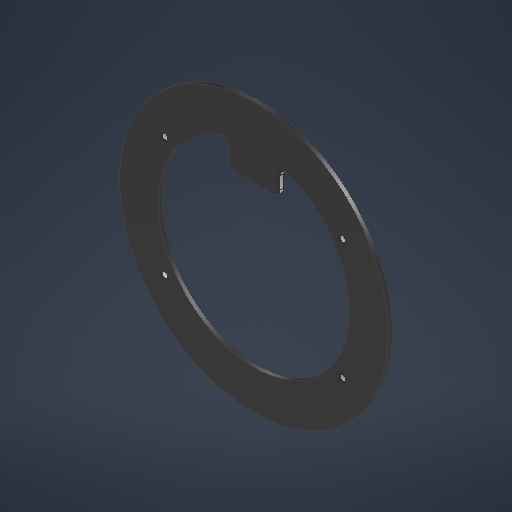
# Autodesk Inventor part: IR Board
Saved by Autodesk Inventor 2026.1 (Build 301233020, 233B)
## iProperties
Created: 2025-11-27
Part Number: IR Board
Material: Generic
Document SubType Name: Modeling
Designer: Bahaa
Density: 1 g/cm^3
Appearance: Default
Mass: 13.7907 g
Surface Area: 152.933 cm^2
Volume: 13.7907 cm^3
Author: Bahaa
Autodesk Inventor part; units mm, degrees
ref_plane "YZ Plane" through (0, 0, 0) normal (1, 0, 0) x (0, 1, 0)
ref_plane "XZ Plane" through (0, 0, 0) normal (0, 1, 0) x (-1, 0, 0)
ref_plane "XY Plane" through (0, 0, 0) normal (0, 0, 1) x (1, 0, 0)
sketch "Sketch1" plane through (0, 0, 0) normal (0, 1, 0) x (-1, 0, 0)
  circle A0 centre (0, 0) radius 65
  line L0 (0, 0) -> (65, 0) construction
  line L1 (0, 0) -> (0, -65) construction
  circle A1 centre (0, 0) radius 46.25
  line L2 (0, 46.25) -> (0, 31.25)
  line L3 (0, 31.25) -> (-34.0955, 31.25)
  line L4 (0, 31.25) -> (34.0955, 31.25)
  line L5 (0, 0) -> (65, 0) construction
  line L6 (0, 0) -> (-46.25, 0) construction
  circle A2 centre (29, 43) radius 1.35
  circle A3 centre (-29, 43) radius 1.35
  circle A4 centre (29, -43) radius 1.35
  circle A5 centre (-29, -43) radius 1.35
  circle A6 centre (-43, 29) radius 1.35
  circle A7 centre (-43, -29) radius 1.35
  circle A8 centre (43, 29) radius 1.35
  circle A9 centre (43, -29) radius 1.35
  circle A10 centre (-29, -43) radius 1.35
  circle A11 centre (29, -43) radius 1.35
  circle A12 centre (-29, 43) radius 1.35
  circle A13 centre (29, 43) radius 1.35
  circle A14 centre (43, -29) radius 1.35
  circle A15 centre (43, 29) radius 1.35
  circle A16 centre (-43, -29) radius 1.35
  circle A17 centre (-43, 29) radius 1.35
  line L7 (12.5, 46.25) -> (-12.5, 46.25)
  line L8 (-12.5, 46.25) -> (-12.5, 31.25)
  line L9 (-12.5, 31.25) -> (12.5, 31.25)
  line L10 (12.5, 31.25) -> (12.5, 46.25)
  line L11 (12.5, 46.25) -> (-12.5, 31.25) construction
  line L12 (-12.5, 46.25) -> (12.5, 31.25) construction
  point P0 (0, -46.25)
  point P1 (0, 38.75)
  point P2 (-12.5, 44.5288)
  point P3 (12.5, 44.5288)
  dimension "d0" = 130
  dimension "d18" = 92.5
  dimension "d21" = 62.5
  dimension "d29" = 86
  dimension "d30" = 29
  dimension "d31" = 2.7
  dimension "d47" = 360
  dimension "d49" = 25
  constraints: 26 end point, 18 centre point, 6 coincident, 6 point on circle, 5 symmetric about line, 4 horizontal, 3 midpoint, 2 parallel, 2 perpendicular, 2 point on line, 2 vertical, 1 vertical alignment, 38 other
  measures "d0" diameter of A0
  measures "d18" diameter of A1
  measures "d21" diameter of L3 L0
  measures "d29" diameter of point (29, 43) L0
  measures "d30" horizontal distance of point (0, 0) point (29, 43)
  measures "d31" diameter of A2
  measures "d49" distance of L9.end L8.end
extrude "Extrusion1" add sketch "Sketch1" along normal blind 2 contours A0 | L10 L4 L2 A1 | A1 L7 L10 | L8 L7 A1 | A1 L2 L3 L8 | A2 | A3 | A4 | A5
sketch "Sketch2" plane through (0, 0, 0) normal (0, -1, 0) x (1, 0, 0)
  circle A0 centre (0, 0) radius 65 construction
  line L0 (-4, 55) -> (4, 55)
  line L1 (4, 55) -> (4, 61)
  line L2 (-4, 61) -> (-4, 55)
  line L3 (-4, 55) -> (4, 61) construction
  line L4 (4, 55) -> (-4, 61) construction
  line L5 (0, 0) -> (0, 71.2779) construction
  arc A1 (4, 61) -> (-4, 61) centre (0, 61) ccw
  line L6 (-24.7431, 49.2826) -> (-17.3521, 52.3441)
  line L7 (-17.3521, 52.3441) -> (-19.6482, 57.8874)
  line L8 (-27.0392, 54.8259) -> (-24.7431, 49.2826)
  line L9 (-24.7431, 49.2826) -> (-19.6482, 57.8874) construction
  line L10 (-17.3521, 52.3441) -> (-27.0392, 54.8259) construction
  arc A2 (-19.6482, 57.8874) -> (-27.0392, 54.8259) centre (-23.3437, 56.3567) ccw
  line L11 (-41.7193, 36.0624) -> (-36.0624, 41.7193)
  line L12 (-36.0624, 41.7193) -> (-40.3051, 45.9619)
  line L13 (-45.9619, 40.3051) -> (-41.7193, 36.0624)
  line L14 (-41.7193, 36.0624) -> (-40.3051, 45.9619) construction
  line L15 (-36.0624, 41.7193) -> (-45.9619, 40.3051) construction
  arc A3 (-40.3051, 45.9619) -> (-45.9619, 40.3051) centre (-43.1335, 43.1335) ccw
  line L16 (-52.3441, 17.3521) -> (-49.2826, 24.7431)
  line L17 (-49.2826, 24.7431) -> (-54.8259, 27.0392)
  line L18 (-57.8874, 19.6482) -> (-52.3441, 17.3521)
  line L19 (-52.3441, 17.3521) -> (-54.8259, 27.0392) construction
  line L20 (-49.2826, 24.7431) -> (-57.8874, 19.6482) construction
  arc A4 (-54.8259, 27.0392) -> (-57.8874, 19.6482) centre (-56.3567, 23.3437) ccw
  line L21 (-55, -4) -> (-55, 4)
  line L22 (-55, 4) -> (-61, 4)
  line L23 (-61, -4) -> (-55, -4)
  line L24 (-55, -4) -> (-61, 4) construction
  line L25 (-55, 4) -> (-61, -4) construction
  arc A5 (-61, 4) -> (-61, -4) centre (-61, 0) ccw
  line L26 (-49.2826, -24.7431) -> (-52.3441, -17.3521)
  line L27 (-52.3441, -17.3521) -> (-57.8874, -19.6482)
  line L28 (-54.8259, -27.0392) -> (-49.2826, -24.7431)
  line L29 (-49.2826, -24.7431) -> (-57.8874, -19.6482) construction
  line L30 (-52.3441, -17.3521) -> (-54.8259, -27.0392) construction
  arc A6 (-57.8874, -19.6482) -> (-54.8259, -27.0392) centre (-56.3567, -23.3437) ccw
  line L31 (-36.0624, -41.7193) -> (-41.7193, -36.0624)
  line L32 (-41.7193, -36.0624) -> (-45.9619, -40.3051)
  line L33 (-40.3051, -45.9619) -> (-36.0624, -41.7193)
  line L34 (-36.0624, -41.7193) -> (-45.9619, -40.3051) construction
  line L35 (-41.7193, -36.0624) -> (-40.3051, -45.9619) construction
  arc A7 (-45.9619, -40.3051) -> (-40.3051, -45.9619) centre (-43.1335, -43.1335) ccw
  line L36 (-17.3521, -52.3441) -> (-24.7431, -49.2826)
  line L37 (-24.7431, -49.2826) -> (-27.0392, -54.8259)
  line L38 (-19.6482, -57.8874) -> (-17.3521, -52.3441)
  line L39 (-17.3521, -52.3441) -> (-27.0392, -54.8259) construction
  line L40 (-24.7431, -49.2826) -> (-19.6482, -57.8874) construction
  arc A8 (-27.0392, -54.8259) -> (-19.6482, -57.8874) centre (-23.3437, -56.3567) ccw
  line L41 (4, -55) -> (-4, -55)
  line L42 (-4, -55) -> (-4, -61)
  line L43 (4, -61) -> (4, -55)
  line L44 (4, -55) -> (-4, -61) construction
  line L45 (-4, -55) -> (4, -61) construction
  arc A9 (-4, -61) -> (4, -61) centre (0, -61) ccw
  line L46 (24.7431, -49.2826) -> (17.3521, -52.3441)
  line L47 (17.3521, -52.3441) -> (19.6482, -57.8874)
  line L48 (27.0392, -54.8259) -> (24.7431, -49.2826)
  line L49 (24.7431, -49.2826) -> (19.6482, -57.8874) construction
  line L50 (17.3521, -52.3441) -> (27.0392, -54.8259) construction
  arc A10 (19.6482, -57.8874) -> (27.0392, -54.8259) centre (23.3437, -56.3567) ccw
  line L51 (41.7193, -36.0624) -> (36.0624, -41.7193)
  line L52 (36.0624, -41.7193) -> (40.3051, -45.9619)
  line L53 (45.9619, -40.3051) -> (41.7193, -36.0624)
  line L54 (41.7193, -36.0624) -> (40.3051, -45.9619) construction
  line L55 (36.0624, -41.7193) -> (45.9619, -40.3051) construction
  arc A11 (40.3051, -45.9619) -> (45.9619, -40.3051) centre (43.1335, -43.1335) ccw
  line L56 (52.3441, -17.3521) -> (49.2826, -24.7431)
  line L57 (49.2826, -24.7431) -> (54.8259, -27.0392)
  line L58 (57.8874, -19.6482) -> (52.3441, -17.3521)
  line L59 (52.3441, -17.3521) -> (54.8259, -27.0392) construction
  line L60 (49.2826, -24.7431) -> (57.8874, -19.6482) construction
  arc A12 (54.8259, -27.0392) -> (57.8874, -19.6482) centre (56.3567, -23.3437) ccw
  line L61 (55, 4) -> (55, -4)
  line L62 (55, -4) -> (61, -4)
  line L63 (61, 4) -> (55, 4)
  line L64 (55, 4) -> (61, -4) construction
  line L65 (55, -4) -> (61, 4) construction
  arc A13 (61, -4) -> (61, 4) centre (61, 0) ccw
  line L66 (49.2826, 24.7431) -> (52.3441, 17.3521)
  line L67 (52.3441, 17.3521) -> (57.8874, 19.6482)
  line L68 (54.8259, 27.0392) -> (49.2826, 24.7431)
  line L69 (49.2826, 24.7431) -> (57.8874, 19.6482) construction
  line L70 (52.3441, 17.3521) -> (54.8259, 27.0392) construction
  arc A14 (57.8874, 19.6482) -> (54.8259, 27.0392) centre (56.3567, 23.3437) ccw
  line L71 (36.0624, 41.7193) -> (41.7193, 36.0624)
  line L72 (41.7193, 36.0624) -> (45.9619, 40.3051)
  line L73 (40.3051, 45.9619) -> (36.0624, 41.7193)
  line L74 (36.0624, 41.7193) -> (45.9619, 40.3051) construction
  line L75 (41.7193, 36.0624) -> (40.3051, 45.9619) construction
  arc A15 (45.9619, 40.3051) -> (40.3051, 45.9619) centre (43.1335, 43.1335) ccw
  line L76 (17.3521, 52.3441) -> (24.7431, 49.2826)
  line L77 (24.7431, 49.2826) -> (27.0392, 54.8259)
  line L78 (19.6482, 57.8874) -> (17.3521, 52.3441)
  line L79 (17.3521, 52.3441) -> (27.0392, 54.8259) construction
  line L80 (24.7431, 49.2826) -> (19.6482, 57.8874) construction
  arc A16 (27.0392, 54.8259) -> (19.6482, 57.8874) centre (23.3437, 56.3567) ccw
  point P0 (0, 58)
  point P1 (-22.1956, 53.585)
  point P2 (-41.0122, 41.0122)
  point P3 (-53.585, 22.1956)
  point P4 (-58, 0)
  point P5 (-53.585, -22.1956)
  point P6 (-41.0122, -41.0122)
  point P7 (-22.1956, -53.585)
  point P8 (0, -58)
  point P9 (22.1956, -53.585)
  point P10 (41.0122, -41.0122)
  point P11 (53.585, -22.1956)
  point P12 (58, 0)
  point P13 (53.585, 22.1956)
  point P14 (41.0122, 41.0122)
  point P15 (22.1956, 53.585)
  dimension "d34" = 8
  dimension "d35" = 6
  dimension "d38" = 4
  dimension "d39" = 55
  dimension "d42" = 360
  constraints: 162 end point, 32 point on circle, 16 centre point, 2 midpoint, 2 point on line, 1 horizontal, 1 parallel, 1 perpendicular, 1 vertical, 193 other
  measures "d34" distance of L1.end L2.start
  measures "d35" distance of L1.end L0.end
  measures "d38" radius of A1
  measures "d39" distance from line of point (0, 0) L0
extrude "Extrusion2" [suppressed]
fillet "Fillet1" radius 3 4 edges at (12.5, 1, 44.5288) (12.5, 1, 31.25) (-12.5, 1, 31.25) (-12.5, 1, 44.5288)
body "Solid1"
